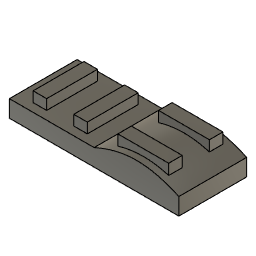
Qatest-Deposition (Autodesk Fusion 360 design; units mm, degrees)
Autodesk Fusion 360 part; units mm, degrees
sketch "Sketch1" plane through (0, 0, 0) normal (0, 1, 0) x (1, 0, 0)
  line L0 (0, -5) -> (0, 0)
  spline S0 degree 5 poles (-25, -5) (-24.5, -5.2275) (-23.5, -5.6628) (-22, -6.256) (-20, -6.9257) (-17.5, -7.5472) (-15, -7.9337) (-12.5, -8.066) (-10, -7.9337) (-7.5, -7.5472) (-5, -6.9257) (-3, -6.256) (-1.5, -5.6628) (-0.5, -5.2275) (0, -5) knots 0 0 0 0 0 0 0.1 0.2 0.3 0.4 0.5 0.6 0.7 0.8 0.9 1 1 1 1 1 1
  line L1 (-25, -5) -> (-50, -5)
  line L2 (-50, -5) -> (-50, 0)
  line L3 (-50, 0) -> (0, 0)
  point P0 (-12.5, -8)
  dimension "d9" = 5
  dimension "d10" = 5
  dimension "d11" = 3
  dimension "d16" = 50
  dimension "d17" = 25
  dimension "d18" = 12.5
  constraint vertical L0
  constraint coincident L0.end L3.end
  constraint horizontal L1
  constraint vertical L2
  constraint perpendicular L0 L3
  measures "d9" distance of L1.end L2.end
  measures "d10" distance of L0.end L0.start
  measures "d11" distance of S0.start P0
  measures "d16" distance of L2.end L0.end
  measures "d17" distance of S0.start L1.end
  measures "d18" distance of S0.start P0
extrude "Extrude1" add sketch "Sketch1" along normal blind 20 makes body 1
ref_plane "WorkPlane1" through (-25, 10, 10) normal (0, 0, -1) x (-1, 0, 0)
sketch "Sketch5" plane through (0, 0, 5) normal (0, 0, 1) x (-1, 0, 0)
  line L0 (50, 0) -> (25, 0)
  line L1 (25, 0) -> (25, -20)
  line L2 (25, -20) -> (50, -20)
  line L3 (50, -20) -> (50, 0)
  line L4 (45.5, -17.5) -> (41.5, -17.5)
  line L5 (41.5, -17.5) -> (41.5, -2.5)
  line L6 (41.5, -2.5) -> (45.5, -2.5)
  line L7 (45.5, -2.5) -> (45.5, -17.5)
  line L8 (33.5, -17.5) -> (29.5, -17.5)
  line L9 (29.5, -17.5) -> (29.5, -2.5)
  line L10 (29.5, -2.5) -> (33.5, -2.5)
  line L11 (33.5, -2.5) -> (33.5, -17.5)
  dimension "d34" = 4
  dimension "d35" = 15
  dimension "d36" = 4
  dimension "d37" = 15
  dimension "d38" = 2.5
  dimension "d39" = 2.5
  dimension "d40" = 8
  dimension "d41" = 4.5
  constraint horizontal L4
  constraint vertical L5
  constraint horizontal L6
  constraint vertical L7
  constraint horizontal L8
  constraint vertical L9
  constraint horizontal L10
  constraint vertical L11
  measures "d34" distance of L4.start L4.end
  measures "d35" distance of L4.start L6.end
  measures "d36" distance of L8.start L8.end
  measures "d37" distance of L8.end L9.end
  measures "d38" distance of L2 L4
  measures "d39" distance of L2 L8
  measures "d40" distance of L5 L11
  measures "d41" distance of L3 L7
extrude "Extrude5" add sketch "Sketch5" along normal blind 3 separate body contours L4 L5 L6 L7 | L8 L9 L10 L11 makes body 2 at (-30.8333, 7.5, 5) makes body 3 at (-42.8333, 7.5, 5)
sketch "Sketch7" plane through (0, 0, 0) normal (0, 0, -1) x (1, 0, 0)
  line L0 (0, 0) -> (-50, 0)
  line L1 (-50, 0) -> (-50, -20)
  line L2 (-50, -20) -> (0, -20)
  line L3 (0, -20) -> (0, 0)
  line L4 (-20, -18) -> (-5, -18)
  line L5 (-5, -18) -> (-5, -14)
  line L6 (-5, -14) -> (-20, -14)
  line L7 (-20, -14) -> (-20, -18)
  line L8 (-20, -6) -> (-5, -6)
  line L9 (-5, -6) -> (-5, -2)
  line L10 (-5, -2) -> (-20, -2)
  line L11 (-20, -2) -> (-20, -6)
  dimension "d44" = 15
  dimension "d45" = 15
  dimension "d46" = 4
  dimension "d47" = 4
  dimension "d48" = 8
  dimension "d49" = 5
  dimension "d50" = 5
  dimension "d51" = 2
  constraint horizontal L4
  constraint vertical L5
  constraint horizontal L6
  constraint vertical L7
  constraint horizontal L8
  constraint vertical L9
  constraint horizontal L10
  constraint vertical L11
  measures "d44" distance of L4.start L4.end
  measures "d45" distance of L8.start L8.end
  measures "d46" distance of L4.end L5.end
  measures "d47" distance of L8.end L9.end
  measures "d48" distance of L6 L8
  measures "d49" distance of L3 L5
  measures "d50" distance of L3 L9
  measures "d51" distance of L0 L10
extrude "Extrude6" add sketch "Sketch7" against normal blind 10 contours L4 L5 L6 L7 | L8 L9 L10 L11 bodies 1
split "Split1" by face at (-3.9286, 4.0952, 6.5401) of body 1 bodies 1 1 makes body 4 at (-15, 15.3333, 10) makes body 5 at (-10, 4.6667, 10)
